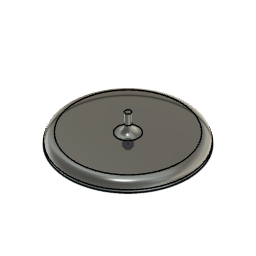
Assembly (Autodesk Fusion 360 archive; units mm, degrees)
design "Base"
Autodesk Fusion 360 part; units mm, degrees
note: some values were not read from the file. Set by a fixed rule: which face or edge a step refers to.
sketch "Sketch1" plane through (0, 0, 0) normal (0, 0, 1) x (1, 0, 0)
  circle A0 centre (0, 0) radius 30
  dimension "d1" = 60
  constraint coincident A0.centre origin
  measures "d1" diameter of A0
extrude "Extrude3" add sketch "Sketch1" along normal blind 5.08
sketch "Sketch2" plane through (0, 0, 5.08) normal (0, 0, 1) x (-1, 0, 0)
  circle A0 centre (0, 0) radius 30
  circle A1 centre (0, 0) radius 1.35
  dimension "d11" = 2.7
  constraint coincident A0.centre A1.centre
  measures "d11" diameter of A1
fillet "Fillet2" radius 3.81 1 edges at (-27.9698, -10.8485, 5.08)
extrude "Extrude4" add sketch "Sketch2" along normal blind 8.89 contours A1
fillet "Fillet3" radius 3.81 1 edges at (1.2586, -0.4882, 5.08)

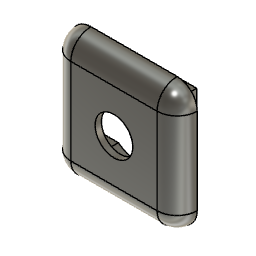
design "Back Plate"
Autodesk Fusion 360 part; units mm, degrees
sketch "Sketch1" plane through (0, 0, 0) normal (0, 1, 0) x (1, 0, 0)
  line L0 (0, 0) -> (69.24, 0)
  line L1 (69.24, 0) -> (69.24, -69.24)
  line L2 (69.24, -69.24) -> (0, -69.24)
  line L3 (0, -69.24) -> (0, 0)
  dimension "d1" = 69.24
  dimension "d2" = 69.24
  constraint horizontal L0
  constraint vertical L1
  constraint horizontal L2
  constraint vertical L3
  constraint coincident L0.start L3.end
  measures "d1" distance of L0.start L0.end
  measures "d2" distance of L0.start L2.end
extrude "Extrude1" add sketch "Sketch1" along normal blind 5.08
sketch "Sketch2" plane through (0, 0, 0) normal (0, -1, 0) x (1, 0, 0)
  line L0 (69.24, 69.24) -> (0, 69.24)
  line L1 (0, 69.24) -> (0, 0)
  line L2 (0, 0) -> (69.24, 0)
  line L3 (69.24, 0) -> (69.24, 69.24)
  line L4 (-5.38, 74.62) -> (74.62, 74.62)
  line L5 (74.62, 74.62) -> (74.62, -5.38)
  line L6 (74.62, -5.38) -> (-5.38, -5.38)
  line L7 (-5.38, -5.38) -> (-5.38, 74.62)
  point P0 (34.62, 69.24)
  point P1 (34.62, 74.62)
  point P2 (0, 34.62)
  point P3 (-5.38, 34.62)
  dimension "d5" = 80
  dimension "d6" = 80
  constraint horizontal L4
  constraint vertical L5
  constraint horizontal L6
  constraint vertical L7
  constraint midpoint L0 P0
  constraint midpoint L4 P1
  constraint vertical P0 P1
  constraint midpoint L1 P2
  constraint midpoint L7 P3
  constraint horizontal P2 P3
  measures "d5" distance of L4.start L4.end
  measures "d6" distance of L4.start L6.end
extrude "Extrude2" add sketch "Sketch2" along normal blind 12.7 contours L0 L1 L2 L3 | L4 L5 L6 L7
fillet "Fillet1" radius 12.7 8 edges at (-5.38, -6.35, 74.62) (74.62, -6.35, 74.62) (74.62, -6.35, -5.38) (-5.38, -6.35, -5.38) (34.62, -12.7, 74.62) (-5.38, -12.7, 34.62) (74.62, -12.7, 34.62) (34.62, -12.7, -5.38)
sketch "Sketch4" plane through (0, -12.7, 0) normal (0, -1, 0) x (1, 0, 0)
  line L0 (7.32, 7.32) -> (61.92, 7.32)
  line L1 (61.92, 7.32) -> (61.92, 61.92)
  line L2 (61.92, 61.92) -> (7.32, 61.92)
  line L3 (7.32, 61.92) -> (7.32, 7.32)
  circle A0 centre (34.62, 34.62) radius 11.938
  dimension "d18" = 23.876
  measures "d18" diameter of A0
extrude "Extrude4" cut sketch "Sketch4" against normal up to surface (17.78 mm away) contours A0
sketch "Sketch5" plane through (0, 5.08, 0) normal (0, 1, 0) x (-1, 0, 0)
  circle A0 centre (-34.62, 34.62) radius 11.938
  line L0 (0, 69.24) -> (-69.24, 69.24)
  line L1 (-69.24, 69.24) -> (-69.24, 0)
  line L2 (-69.24, 0) -> (0, 0)
  line L3 (0, 0) -> (0, 69.24)
  circle A1 centre (-34.62, 34.62) radius 25
  line L4 (-69.24, 54.62) -> (0, 54.62)
  line L5 (0, 54.62) -> (0, 14.62)
  line L6 (0, 14.62) -> (-69.24, 14.62)
  line L7 (-69.24, 14.62) -> (-69.24, 54.62)
  line L8 (-69.24, 54.62) -> (0, 14.62) construction
  line L9 (0, 54.62) -> (-69.24, 14.62) construction
  point P0 (-34.62, 34.62)
  dimension "d21" = 50
  dimension "d24" = 40
  constraint concentric A0 A1
  constraint horizontal L4
  constraint perpendicular L4 L5
  constraint parallel L4 L6
  constraint parallel L5 L7
  constraint coincident L8 P0
  constraint coincident L9 P0
  constraint coincident P0 A0.centre
  measures "d21" diameter of A1
  measures "d24" distance of L4.end L5.end
extrude "Extrude5" cut sketch "Sketch5" against normal blind 13.78 contours L3 A1 L4 L5 L6 | L1 A1 L4 L6 L7 | A1 L4 | A1 L4 L6 | A1 L6
ref_plane "WorkPlane2" through (34.62, 2.54, -7.62) normal (0, 0, -1) x (-1, 0, 0)
sketch "Sketch7" plane through (0, 0, -7.62) normal (0, 0, -1) x (-1, 0, 0)
  line L0 (-61.92, 0) -> (-7.32, 0)
  circle A0 centre (-34.62, 0) radius 5.08
  dimension "d28" = 10.16
  constraint midpoint L0 A0.centre
  measures "d28" diameter of A0
extrude "Extrude6" cut sketch "Sketch7" against normal blind 5.08 contours L0 A0 picked at (-34.2432, -1.6509)
equation "d1 = 8 cm - 0.4 in - 0.6 mm"
equation "d2 = 8 cm - 0.4 in - 0.6 mm"
equation "d22 = -( 0.7 in - 0.4 cm )"

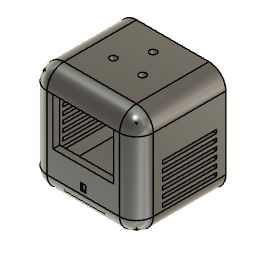
design "Cube"
Autodesk Fusion 360 part; units mm, degrees
sketch "Sketch1" plane through (0, 0, 0) normal (0, 0, 1) x (1, 0, 0)
  line L0 (0, 0) -> (80, 0)
  line L1 (80, 0) -> (80, 80)
  line L2 (80, 80) -> (0, 80)
  line L3 (0, 80) -> (0, 0)
  dimension "d1" = 80
  dimension "d2" = 80
  constraint horizontal L0
  constraint vertical L1
  constraint horizontal L2
  constraint vertical L3
  constraint coincident L0.start L3.end
  measures "d1" distance of L0.start L0.end
  measures "d2" distance of L0.start L2.end
extrude "Extrude1" add sketch "Sketch1" along normal blind 80
sketch "Sketch2" plane through (0, 0, 0) normal (0, -1, 0) x (1, 0, 0)
  line L0 (0, 0) -> (80, 0)
  line L1 (80, 0) -> (80, 80)
  line L2 (80, 80) -> (0, 80)
  line L3 (0, 80) -> (0, 0)
  circle A0 centre (40, 40) radius 4.9498
  dimension "d5" = 9.8996
  measures "d5" diameter of A0
shell "Shell1" thickness 5.08 removed faces 1 at (53.3333, 80, 26.6667)
sketch "Sketch4" plane through (0, 0, 0) normal (0, 0, -1) x (1, 0, 0)
  line L0 (0, 0) -> (0, -80)
  line L1 (0, -80) -> (80, -80)
  line L2 (80, -80) -> (80, 0)
  line L3 (80, 0) -> (0, 0)
  circle A0 centre (40, -40) radius 3.65
  dimension "d10" = 7.3
  measures "d10" diameter of A0
extrude "Extrude3" cut sketch "Sketch4" against normal up to surface (5.08 mm away) contours A0
sketch "Sketch5" plane through (0, 0, 80) normal (0, 0, 1) x (-1, 0, 0)
  line L0 (0, -80) -> (0, 0)
  line L1 (0, 0) -> (-80, 0)
  line L2 (-80, 0) -> (-80, -80)
  line L3 (-80, -80) -> (0, -80)
  circle A0 centre (-40, -40) radius 12.7
  circle A1 centre (-40, -52.7) radius 2.54
  circle A2 centre (-29.0015, -33.65) radius 2.54
  circle A3 centre (-50.9985, -33.65) radius 2.54
  dimension "d13" = 25.4
  dimension "d14" = 5.08
  dimension "d16" = 360
  constraint coincident A0 A1.centre
  measures "d13" diameter of A0
  measures "d14" diameter of A1
extrude "Extrude4" cut sketch "Sketch5" against normal up to surface (5.08 mm away) contours A0 A2 | A0 A2 | A0 A1 | A0 A1 | A0 A3 | A0 A3
sketch "Sketch8" plane through (0, 0, 0) normal (0, -1, 0) x (1, 0, 0)
  line L0 (0, 0) -> (80, 0)
  line L1 (80, 0) -> (80, 80)
  line L2 (80, 80) -> (0, 80)
  line L3 (0, 80) -> (0, 0)
  line L4 (17.14, 67.3) -> (62.86, 67.3)
  line L5 (62.86, 67.3) -> (62.86, 31.74)
  line L6 (62.86, 31.74) -> (17.14, 31.74)
  line L7 (17.14, 31.74) -> (17.14, 67.3)
  line L8 (41.905, 20.32) -> (38.095, 20.32)
  line L9 (38.095, 20.32) -> (38.095, 15.24)
  line L10 (38.095, 15.24) -> (41.905, 15.24)
  line L11 (41.905, 15.24) -> (41.905, 20.32)
  line L12 (41.905, 20.32) -> (38.095, 15.24) construction
  line L13 (38.095, 20.32) -> (41.905, 15.24) construction
  line L14 (5.08, 5.08) -> (74.92, 5.08)
  point P0 (40, 17.78)
  dimension "d38" = 45.72
  dimension "d39" = 35.56
  dimension "d40" = 3.81
  dimension "d41" = 5.08
  dimension "d42" = 10.16
  dimension "d43" = 40
  dimension "d44" = 17.14
  dimension "d45" = 12.7
  constraint horizontal L4
  constraint vertical L5
  constraint horizontal L6
  constraint vertical L7
  constraint horizontal L8
  constraint perpendicular L8 L9
  constraint parallel L8 L10
  constraint parallel L9 L11
  constraint coincident L12 P0
  constraint coincident L13 P0
  measures "d38" distance of L4.start L4.end
  measures "d39" distance of L4.start L6.end
  measures "d40" distance of L9.end L10.end
  measures "d41" distance of L8.end L9.end
  measures "d42" distance of L10 L14
  measures "d43" distance of L1 P0
  measures "d44" distance of L1 L5
  measures "d45" distance of L2 L4
extrude "Extrude7" cut sketch "Sketch8" against normal up to surface (5.08 mm away) contours L4 L5 L6 L7 | L8 L9 L10 L11
sketch "Sketch9" plane through (80, 0, 0) normal (1, 0, 0) x (0, 1, 0)
  line L0 (0, 0) -> (80, 0)
  line L1 (80, 0) -> (80, 80)
  line L2 (80, 80) -> (0, 80)
  line L3 (0, 80) -> (0, 0)
  line L4 (19.68, 17.78) -> (60.32, 17.78)
  line L5 (60.32, 17.78) -> (60.32, 15.24)
  line L6 (60.32, 15.24) -> (19.68, 15.24)
  line L7 (19.68, 15.24) -> (19.68, 17.78)
  line L8 (60.32, 23.368) -> (60.32, 20.828)
  line L9 (19.68, 23.368) -> (60.32, 23.368)
  line L10 (19.68, 20.828) -> (19.68, 23.368)
  line L11 (60.32, 20.828) -> (19.68, 20.828)
  line L12 (60.32, 28.956) -> (60.32, 26.416)
  line L13 (19.68, 28.956) -> (60.32, 28.956)
  line L14 (19.68, 26.416) -> (19.68, 28.956)
  line L15 (60.32, 26.416) -> (19.68, 26.416)
  line L16 (60.32, 34.544) -> (60.32, 32.004)
  line L17 (19.68, 34.544) -> (60.32, 34.544)
  line L18 (19.68, 32.004) -> (19.68, 34.544)
  line L19 (60.32, 32.004) -> (19.68, 32.004)
  line L20 (60.32, 40.132) -> (60.32, 37.592)
  line L21 (19.68, 40.132) -> (60.32, 40.132)
  line L22 (19.68, 37.592) -> (19.68, 40.132)
  line L23 (60.32, 37.592) -> (19.68, 37.592)
  line L24 (60.32, 45.72) -> (60.32, 43.18)
  line L25 (19.68, 45.72) -> (60.32, 45.72)
  line L26 (19.68, 43.18) -> (19.68, 45.72)
  line L27 (60.32, 43.18) -> (19.68, 43.18)
  dimension "d48" = 40.64
  dimension "d50" = 19.68
  dimension "d51" = 15.24
  dimension "d55" = 2.54
  dimension "d58" = 0
  dimension "d59" = 27.94
  constraint horizontal L4
  constraint vertical L5
  constraint horizontal L6
  constraint vertical L7
  measures "d48" distance of L4.start L4.end
  measures "d50" distance of L1 L5
  measures "d51" distance of L0 L6
  measures "d55" distance of L4.start L6.end
extrude "Extrude8" cut sketch "Sketch9" against normal blind 88.9 contours L4 L5 L6 L7
extrude "Extrude9" cut sketch "Sketch9" against normal blind 86.36 contours L8 L9 L10 L11 | L12 L13 L14 L15 | L16 L17 L18 L19 | L20 L21 L22 L23 | L24 L25 L26 L27
sketch "Sketch10" plane through (0, 80, 0) normal (0, 1, 0) x (-1, 0, 0)
  line L0 (-80, 80) -> (-80, 0)
  line L1 (-80, 0) -> (0, 0)
  line L2 (0, 0) -> (0, 80)
  line L3 (-5.08, 74.92) -> (-5.08, 5.08)
  line L4 (-5.08, 5.08) -> (-74.92, 5.08)
  line L5 (-74.92, 5.08) -> (-74.92, 74.92)
  line L6 (-74.92, 74.92) -> (-5.08, 74.92)
  line L7 (0, 80) -> (-80, 80)
  line L8 (-74.92, 74.92) -> (-5.08, 74.92)
  line L9 (-5.08, 74.92) -> (-5.08, 5.08)
  line L10 (-5.08, 5.08) -> (-74.92, 5.08)
  line L11 (-74.92, 5.08) -> (-74.92, 74.92)
  constraint horizontal L8
  constraint vertical L9
  constraint horizontal L10
  constraint vertical L11
  constraint coincident L3.end L4.start
  constraint coincident L5.end L6.start
extrude "Extrude10" add sketch "Sketch10" against normal blind 5.08 contours L3 L4 L5 L6 L8 L9 L10 L11
fillet "Fillet2" radius 12.7 12 edges at (80, 40, 80) (40, 80, 80) (80, 80, 40) (0, 80, 40) (0, 40, 80) (40, 80, 0) (80, 40, 0) (80, 0, 40) (0, 40, 0) (40, 0, 0) (0, 0, 40) (40, 0, 80)
sketch "Sketch13" plane through (0, 80, 0) normal (0, 1, 0) x (-1, 0, 0)
  line L0 (-67.3, 67.3) -> (-67.3, 12.7)
  line L1 (-67.3, 12.7) -> (-12.7, 12.7)
  line L2 (-12.7, 12.7) -> (-12.7, 67.3)
  line L3 (-12.7, 67.3) -> (-67.3, 67.3)
  line L4 (-88.9, 88.9) -> (12.7, 88.9)
  line L5 (12.7, 88.9) -> (12.7, -12.7)
  line L6 (12.7, -12.7) -> (-88.9, -12.7)
  line L7 (-88.9, -12.7) -> (-88.9, 88.9)
  constraint horizontal L4
  constraint vertical L5
  constraint horizontal L6
  constraint vertical L7
extrude "Extrude12" cut sketch "Sketch13" against normal blind 12.7 contours L0 L1 L2 L3 | L4 L5 L6 L7
sketch "Sketch14" plane through (0, 5.08, 0) normal (0, 1, 0) x (-1, 0, 0)
  line L0 (-17.14, 67.3) -> (-17.14, 31.74)
  line L1 (-17.14, 31.74) -> (-62.86, 31.74)
  line L2 (-62.86, 31.74) -> (-62.86, 67.3)
  line L3 (-62.86, 67.3) -> (-17.14, 67.3)
  line L4 (-38.095, 15.24) -> (-41.905, 15.24)
  line L5 (-41.905, 15.24) -> (-41.905, 20.32)
  line L6 (-41.905, 20.32) -> (-38.095, 20.32)
  line L7 (-38.095, 20.32) -> (-38.095, 15.24)
  line L8 (-74.92, 5.08) -> (-5.08, 5.08)
  line L9 (-5.08, 5.08) -> (-5.08, 74.92)
  line L10 (-5.08, 74.92) -> (-74.92, 74.92)
  line L11 (-74.92, 74.92) -> (-74.92, 5.08)
  line L12 (-25, 27.78) -> (-55, 27.78)
  line L13 (-55, 27.78) -> (-55, 7.78)
  line L14 (-55, 7.78) -> (-25, 7.78)
  line L15 (-25, 7.78) -> (-25, 27.78)
  line L16 (-25, 27.78) -> (-55, 7.78) construction
  line L17 (-55, 27.78) -> (-25, 7.78) construction
  point P0 (-40, 17.78)
  dimension "d73" = 30
  dimension "d74" = 20
  constraint horizontal L12
  constraint perpendicular L12 L13
  constraint parallel L12 L14
  constraint parallel L13 L15
  constraint coincident L16 P0
  constraint coincident L17 P0
  measures "d73" distance of L13.end L14.end
  measures "d74" distance of L12.end L13.end
extrude "Extrude13" cut sketch "Sketch14" against normal blind 3.81 contours L12 L13 L14 L15
equation "d5 = 0.374 in + 0.4 mm"
equation "d44 = ( 8 cm - 1.8 in ) / 2"
equation "d50 = ( 8 cm - 1.6 in ) / 2"

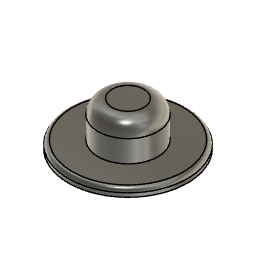
design "Hat"
Autodesk Fusion 360 part; units mm, degrees
sketch "Sketch2" plane through (0, 0, 0) normal (0, 0, 1) x (1, 0, 0)
  circle A0 centre (0, 0) radius 38.1
  dimension "d15" = 76.2
  constraint coincident A0.centre origin
  measures "d15" diameter of A0
extrude "Extrude1" add sketch "Sketch2" along normal blind 5
sketch "Sketch3" plane through (0, 0, 5) normal (0, 0, 1) x (-1, 0, 0)
  circle A0 centre (0, 0) radius 38.1
  circle A1 centre (0, 0) radius 19.05
  dimension "d14" = 38.1
  constraint concentric A0 A1
  measures "d14" diameter of A1
extrude "Extrude2" add sketch "Sketch3" along normal blind 22.86 contours A1
sketch "Sketch4" plane through (0, 0, 0) normal (0, 0, -1) x (1, 0, 0)
  circle A0 centre (0, 0) radius 38.1
  circle A1 centre (0.0969, -12.6996) radius 2.2098
  circle A2 centre (10.9498, 6.4337) radius 2.2098
  circle A3 centre (-11.0466, 6.2659) radius 2.2098
  arc A4 (2.2968, -12.4906) -> (11.8992, 4.4383) centre (0, 0) ccw
  arc A5 (9.6688, 8.2343) -> (-9.7933, 8.0859) centre (0, 0) ccw
  arc A6 (-11.9656, 4.2562) -> (-2.106, -12.5242) centre (0, 0) ccw
  dimension "d7" = 4.4196
  dimension "d9" = 360
  constraint coincident A0.centre A4.centre
  constraint coincident A1.centre A4
  constraint coincident A1 A6.end
  constraint coincident A1 A4.start
  constraint coincident A2 A4.end
  constraint coincident A2 A5.start
  constraint concentric A4 A5
  constraint coincident A3 A5.end
  constraint coincident A3 A6.start
  constraint concentric A5 A6
  measures "d7" diameter of A1
extrude "Extrude3" add sketch "Sketch4" along normal blind 5 contours A1 | A2 | A3
fillet "Fillet2" radius 8.89 1 edges at (17.7608, 6.8888, 27.86)
fillet "Fillet3" radius 2.54 1 edges at (-35.5217, -13.7775, 5)

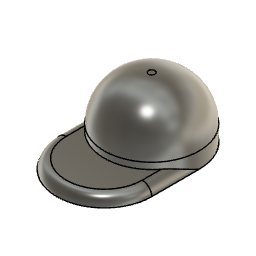
design "Cap"
Autodesk Fusion 360 part; units mm, degrees
sketch "Sketch2" plane through (0, 0, 0) normal (0, 0, 1) x (1, 0, 0)
  circle A0 centre (0, 0) radius 19.05
  dimension "d15" = 38.1
  constraint coincident A0.centre origin
  measures "d15" diameter of A0
extrude "Extrude1" add sketch "Sketch2" along normal blind 20.32
fillet "Fillet4" radius 17.78 1 edges at (-17.7608, -6.8888, 20.32)
sketch "Sketch5" plane through (0, 0, 0) normal (0, 0, -1) x (1, 0, 0)
  circle A0 centre (0, 19.05) radius 19.05
  line L0 (19.05, 0) -> (19.05, 19.05)
  line L1 (-19.05, 0) -> (-19.05, 19.05)
  circle A1 centre (0, 0) radius 19.05
  dimension "d22" = 38.1
  constraint coincident A0 L0.end
  constraint tangent A0 L0
  constraint vertical L0
  constraint coincident A0 L1.end
  constraint tangent A0 L1
  constraint vertical L1
  measures "d22" diameter of A0
extrude "Extrude4" add sketch "Sketch5" along normal blind 3.81
sketch "Sketch6" plane through (0, 0, -3.81) normal (0, 0, -1) x (1, 0, 0)
  line L0 (19.05, 0) -> (19.05, 19.05)
  arc A0 (19.05, 19.05) -> (-19.05, 19.05) centre (0, 19.05) ccw
  line L1 (-19.05, 19.05) -> (-19.05, 0)
  arc A1 (-19.05, 0) -> (19.05, 0) centre (0, 0) ccw
  circle A2 centre (0, 0) radius 12.7
  circle A3 centre (0, -12.7) radius 2.2098
  circle A4 centre (10.9985, 6.35) radius 2.2098
  circle A5 centre (-10.9985, 6.35) radius 2.2098
  dimension "d28" = 25.4
  dimension "d29" = 4.4196
  dimension "d31" = 360
  constraint concentric A1 A2
  constraint coincident A2 A3.centre
  measures "d28" diameter of A2
  measures "d29" diameter of A3
extrude "Extrude5" add sketch "Sketch6" along normal blind 5 contours A2 A4 | A2 A4 | A2 A3 | A2 A3 | A2 A5 | A2 A5
fillet "Fillet5" radius 3.81 3 edges at (19.05, -9.525, 0) (0, -38.1, 0) (-19.05, -9.525, 0)

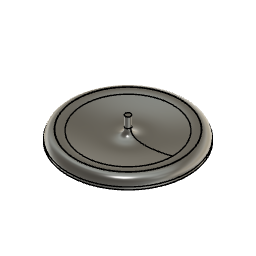
design "New Base"
Autodesk Fusion 360 part; units mm, degrees
sketch "Sketch1" plane through (0, 0, 0) normal (0, 1, 0) x (1, 0, 0)
  line L0 (0, 0) -> (30, 0)
  line L1 (30, 0) -> (30, -1.27)
  line L2 (0, 0) -> (0, -11.43)
  line L3 (0, -11.43) -> (1.35, -11.43)
  line L4 (1.35, -11.43) -> (1.35, -6.35)
  spline S0 degree 5 poles (1.35, -6.35) (1.35, -5.9694) (1.4278, -5.2602) (1.778, -4.3531) (2.6877, -3.4451) (4.4374, -2.753) (6.6502, -2.4321) (9.1882, -2.411) (11.9484, -2.6271) (14.8581, -3.0298) (17.5367, -3.5208) (19.6582, -3.9761) (21.1842, -4.334) (22.0932, -4.5575) (22.3741, -4.6275) knots 0 0 0 0 0 0 0.1 0.2 0.3 0.4 0.5 0.6 0.7 0.8 0.9 0.944585 0.944585 0.944585 0.944585 0.944585 0.944585
  line L5 (26.19, -5.08) -> (26.0602, -5.08)
  arc A0 (26.19, -5.08) -> (30, -1.27) centre (26.19, -1.27) ccw
  arc A1 (22.3741, -4.6275) -> (26.0602, -5.08) centre (26.0602, 10.16) ccw
  point P0 (30, -5.08)
  point P1 (6.35, -2.54)
  dimension "d1" = 30
  dimension "d2" = 5.08
  dimension "d3" = 11.43
  dimension "d4" = 1.35
  dimension "d5" = 5.08
  dimension "d6" = 3.81
  dimension "d7" = 15.24
  constraint coincident L0.start L2.start
  constraint horizontal L0
  constraint perpendicular L0 L1
  constraint perpendicular L0 L2
  constraint perpendicular L2 L3
  constraint perpendicular L3 L4
  constraint coincident P0 L5
  constraint coincident P0 L1
  constraint tangent L5 A0
  constraint tangent L1 A0
  constraint tangent S0 A1
  constraint tangent L5 A1
  measures "d1" distance of L0.start L0.end
  measures "d2" distance of L0.end P0
  measures "d3" distance of L0.start L2.end
  measures "d4" distance of L2.end L3.end
  measures "d5" distance of L3.end L4.end
  measures "d6" radius of A0
  measures "d7" radius of A1
revolve "Revolve1" add sketch "Sketch1" angle 360 about axis through (0, 0, 0) along (0, 0, 1)
equation "d4 = 2.7 mm / 2"
